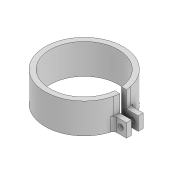
# Autodesk Inventor part: Bearing_fixing
Saved by Autodesk Inventor 2022 (Build 260153000, 153)
## iProperties
Created: 2022-07-04
Part Number: Bearing_fixing
Material: Generic
Document SubType Name: Modeling
Designer: dell
Density: 1 g/cm^3
Appearance: Default
Author: dell
Autodesk Inventor part; units mm, degrees
ref_plane "YZ Plane" through (0, 0, 0) normal (1, 0, 0) x (0, 1, 0)
ref_plane "XZ Plane" through (0, 0, 0) normal (0, 1, 0) x (-1, 0, 0)
ref_plane "XY Plane" through (0, 0, 0) normal (0, 0, 1) x (1, 0, 0)
sketch "Sketch1" plane through (0, 0, 0) normal (0, 1, 0) x (-1, 0, 0)
  circle A0 centre (0, 0) radius 20.25
  circle A1 centre (0, 0) radius 23.25
  line L0 (-20.151, 2) -> (-30.151, 2)
  line L1 (-30.151, 2) -> (-30.151, 5)
  line L2 (-30.151, 5) -> (-20.151, 5)
  line L3 (-20.151, 5) -> (-20.151, 2)
  line L4 (-20.151, -2) -> (-30.151, -2)
  line L5 (-30.151, -2) -> (-30.151, -5)
  line L6 (-30.151, -5) -> (-20.151, -5)
  line L7 (-20.151, -5) -> (-20.151, -2)
  point P0 (-22.706, -5)
  point P1 (-22.706, 5)
  dimension "d0" = 40.5
  dimension "d2" = 3
  dimension "d3" = 3
  dimension "d4" = 2
  dimension "d5" = 10
  dimension "d17" = 3
  constraints: 16 end point, 4 parallel, 2 centre point, 2 horizontal, 2 perpendicular, 2 point on circle, 2 point on line, 1 coincident
  measures "d0" diameter of A0
  measures "d2" distance of L0.end L1.end
  measures "d3" distance of L4.end L5.end
  measures "d4" distance from line of point (0, 0) L0
  measures "d5" distance between parallel lines of L3 L1
  measures "d17" radial gap between concentric circles of A1 A0
extrude "Extrusion1" add sketch "Sketch1" along normal blind 18 contours A0 L3 L2 A1 L6 L7 | L0 A1 L2 L3 | L7 L6 A1 L4 | L0 L1 L2 A1 | A1 L6 L5 L4
sketch "Sketch2" plane through (0, 18, 0) normal (0, 1, 0) x (1, 0, 0)
  line L0 (22.706, -5) -> (30.151, -5) projected
  line L1 (30.151, -5) -> (30.151, -2) projected
  line L2 (30.151, -2) -> (20.151, -2) projected
  arc A0 (20.151, 2) -> (20.151, -2) centre (0, 0) ccw projected
  line L3 (20.151, 2) -> (30.151, 2) projected
  line L4 (30.151, 2) -> (30.151, 5) projected
  line L5 (30.151, 5) -> (22.706, 5) projected
  arc A1 (22.706, 5) -> (22.706, -5) centre (0, 0) ccw projected
  line L6 (22.706, -5) -> (30.151, -5) projected
  arc A2 (22.706, -5) -> (22.706, 5) centre (0, 0) ccw
  point P0 (23.1638, -2)
  point P1 (23.1638, 2)
  constraints: 2 point on circle, 1 centre point, 1 equal radius
extrude "Extrusion2" cut sketch "Sketch2" against normal blind 10 contours A2 L2 L1 L0 | L5 L4 L3 A2
sketch "Sketch3" plane through (22.706, 0, 5) normal (0, 0, 1) x (1, 0, 0)
  circle A0 centre (4.0681, 4) radius 1.6
  line L0 (0, 0) -> (7.445, 0) projected
  line L1 (7.445, 8) -> (0, 8) projected
  point P0 (-22.706, 0)
  dimension "d11" = 3.2
  dimension "d12" = 4
  constraints: 1 centre point
  measures "d11" diameter of A0
  measures "d12" distance from line of L0 A0.centre
extrude "Extrusion3" cut sketch "Sketch3" against normal blind 22
fillet "Fillet1" radius 2 2 edges at (22.706, 4, 5) (22.706, 4, -5)
body "Solid1"
